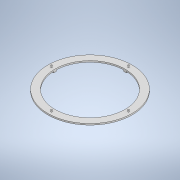
# Autodesk Inventor part: ayudasoporte
Saved by Autodesk Inventor 2021 (Build 250183000, 183)
## iProperties
Created: 2021-09-29
Part Number: ayudasoporte
Material: Genérico
Document SubType Name: Modeling
Designer: orgyn
Density: 1 g/cm^3
Appearance: Valor por defecto
Author: orgyn
Autodesk Inventor part; units mm, degrees
ref_plane "YZ Plane" through (0, 0, 0) normal (1, 0, 0) x (0, 1, 0)
ref_plane "XZ Plane" through (0, 0, 0) normal (0, 1, 0) x (-1, 0, 0)
ref_plane "XY Plane" through (0, 0, 0) normal (0, 0, 1) x (1, 0, 0)
sketch "Boceto1" plane through (0, 0, 0) normal (0, 1, 0) x (-1, 0, 0)
  circle A0 centre (0, 0) radius 60
  circle A1 centre (0, 0) radius 50
  line L0 (0, 0) -> (0, -60)
  line L1 (0, -60) -> (0, -50)
  circle A2 centre (0, -55) radius 1.15
  dimension "d0" = 120
  dimension "d1" = 100
  dimension "d2" = 2.3
  constraints: 4 end point, 2 coincident, 2 vertical alignment, 1 centre point, 1 midpoint, 1 point on line, 1 vertical, 4 other
  measures "d2" diameter of A2
extrude "Extrusión1" add sketch "Boceto1" along normal blind 2 contours A2 L0 | L0 A2 | A0
sketch "Boceto2" plane through (0, 2, 0) normal (0, 1, 0) x (1, 0, 0)
  circle A0 centre (0, 0) radius 50 projected
  line L0 (0, 50) -> (0, 60)
  circle A1 centre (0, 0) radius 60 projected
  circle A2 centre (0, 55) radius 1.15
  circle A3 centre (-55, 0) radius 1.15
  circle A4 centre (0, -55) radius 1.15
  circle A5 centre (55, 0) radius 1.15
  dimension "d5" = 2.3
  dimension "d8" = 360
  constraints: 4 centre point, 2 end point, 2 vertical alignment, 1 midpoint, 1 vertical, 11 other
  measures "d5" diameter of A2
extrude "Extrusión2" add sketch "Boceto2" along normal blind 2 contours A2 L0 | L0 A2 | A3 | A4 | A5
sketch "Boceto3" plane through (0, 0, 0) normal (0, -1, 0) x (1, 0, 0)
  circle A0 centre (0, 0) radius 50 projected
  line L0 (-50, 0) -> (50, 0)
  arc A1 (-50.04, -1.9996) -> (-49.96, -1.9996) centre (-50, 0) ccw
  line L1 (-50.04, -1.9996) -> (-49.96, -1.9996)
  line L2 (-49.96, -1.9996) -> (-52.96, -1.9996)
  line L3 (-52.96, -1.9996) -> (-52.96, 2.2646)
  line L4 (-49.96, 1.9996) -> (-52.96, 2.0596)
  circle A2 centre (0, 0) radius 50
  line L5 (-28.2117, 44.8649) -> (-24.5188, 46.997)
  line L6 (-23.2483, 44.2664) -> (-24.6963, 46.8945)
  line L7 (-26.7117, 42.2668) -> (-28.2117, 44.8649)
  line L8 (24.7483, 46.8645) -> (28.4412, 44.7324)
  line L9 (26.7117, 42.2668) -> (28.2637, 44.8349)
  line L10 (23.2483, 44.2664) -> (24.7483, 46.8645)
  line L11 (52.96, 1.9996) -> (52.96, -2.2646)
  line L12 (49.96, -1.9996) -> (52.96, -2.0596)
  line L13 (49.96, 1.9996) -> (52.96, 1.9996)
  line L14 (28.2117, -44.8649) -> (24.5188, -46.997)
  line L15 (23.2483, -44.2664) -> (24.6963, -46.8945)
  line L16 (26.7117, -42.2668) -> (28.2117, -44.8649)
  line L17 (-24.7483, -46.8645) -> (-28.4412, -44.7324)
  line L18 (-26.7117, -42.2668) -> (-28.2637, -44.8349)
  line L19 (-23.2483, -44.2664) -> (-24.7483, -46.8645)
  line L20 (1.9996, -49.96) -> (1.9996, -52.96)
  line L21 (1.9996, -52.96) -> (-2.2646, -52.96)
  line L22 (-1.9996, -49.96) -> (-2.0596, -52.96)
  line L23 (49.96, 1.9996) -> (52.96, 1.9996)
  line L24 (52.96, 1.9996) -> (52.96, -2.2646)
  line L25 (49.96, -1.9996) -> (52.96, -2.0596)
  line L26 (-1.9996, 49.96) -> (-1.9996, 52.96)
  line L27 (-1.9996, 52.96) -> (2.2646, 52.96)
  line L28 (1.9996, 49.96) -> (2.0596, 52.96)
  point P0 (-52.96, 1.9996)
  point P1 (-24.7483, 46.8645)
  point P2 (-26.7517, 42.3361)
  point P3 (28.2117, 44.8649)
  point P4 (23.2883, 44.3357)
  point P5 (52.96, -1.9996)
  point P6 (50.04, 1.9996)
  point P7 (24.7483, -46.8645)
  point P8 (26.7517, -42.3361)
  point P9 (-28.2117, -44.8649)
  point P10 (-23.2883, -44.3357)
  point P11 (1.9996, -50.04)
  point P12 (-1.9996, -52.96)
  point P13 (50.04, 1.9996)
  point P14 (52.96, -1.9996)
  point P15 (-1.9996, 50.04)
  point P16 (1.9996, 52.96)
  dimension "d13" = 3
  dimension "d14" = 100
  dimension "d17" = 360
  dimension "d21" = 360
  constraints: 58 end point, 28 point on line, 6 point on circle, 2 centre point, 2 coincident, 1 horizontal, 1 perpendicular, 1 tangent, 102 other
  measures "d13" distance of L1.end L2.end
  measures "d14" diameter of A2
extrude "Extrusión3" add sketch "Boceto3" along normal blind 2 contours A0 L13 L11 L12 | A0 A1 L2 L3 L4 | A0 L26 L27 L28 | L20 L21 L22 A0
